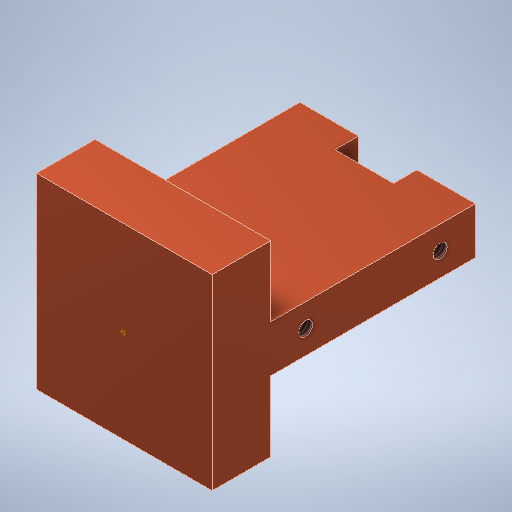
# Autodesk Inventor part: copper_thermal_contact
Saved by Autodesk Inventor 2025 (Build 290162000, 162)
## iProperties
Created: 2024-04-25
Part Number: copper_thermal_contact
Material: Copper
Document SubType Name: Modeling
Designer: warke
Density: 8.94 g/cm^3
Appearance: Copper - Satin
Author: warke
Autodesk Inventor part; units mm, degrees
ref_plane "YZ Plane" through (0, 0, 0) normal (1, 0, 0) x (0, 1, 0)
ref_plane "XZ Plane" through (0, 0, 0) normal (0, 1, 0) x (-1, 0, 0)
ref_plane "XY Plane" through (0, 0, 0) normal (0, 0, 1) x (1, 0, 0)
sketch "Sketch1" plane through (0, 0, 0) normal (0, 1, 0) x (-1, 0, 0)
  line L0 (-7.5, 15) -> (7.5, 15)
  line L1 (7.5, 15) -> (7.5, -15)
  line L2 (7.5, -15) -> (-7.5, -15)
  line L3 (-7.5, -15) -> (-7.5, 15)
  line L4 (-7.5, 15) -> (7.5, -15) construction
  line L5 (7.5, 15) -> (-7.5, -15) construction
  point P0 (0, 0)
  dimension "d0" = 15
  dimension "d1" = 30
  constraints: 12 end point, 2 midpoint, 2 parallel, 1 horizontal, 1 perpendicular
  measures "d0" distance of L1.end L2.end
  measures "d1" distance of L0.end L1.end
extrude "Extrusion1" add sketch "Sketch1" along normal blind 4
chamfer "Chamfer1" distance 2.5 distance2 1 1 edges at (7.5, 2, -15) measured on face at (7.5, 1.3333, 5)
chamfer "Chamfer2" distance 1 distance2 2.5 1 edges at (-7.5, 2, -15) measured on face at (1.8333, 2.6667, -15)
sketch "Sketch3" plane through (0, 0, 0) normal (0, -1, 0) x (1, 0, 0)
  line L0 (0, 0) -> (4, 0)
  line L1 (0, 0) -> (-4, 0)
  dimension "d14" = 4
  dimension "d15" = 4
  constraints: 4 end point, 2 coincident, 2 horizontal
  measures "d14" distance of L0.start L0.end
  measures "d15" distance of L0.start L1.end
hole "Hole1" at (4, 0, 0) at (-4, 0, 0) direction (0, 1, 0) diameter 2.1565 depth 2 thread size "4-40 UNC" class "2B" standard "ANSI Unified Screw Threads"
sketch "Sketch4" plane through (0, 0, 0) normal (0, -1, 0) x (1, 0, 0)
  line L0 (7.5, 15) -> (7.5, -12.5) projected
  line L1 (7.5, -12.5) -> (7.5, -7.5)
  line L2 (7.5, -7.5) -> (2.5, -7.5)
  line L3 (2.5, -7.5) -> (2.5, -5.5)
  line L4 (2.5, -5.5) -> (-2.5, -5.5)
  line L5 (-2.5, -5.5) -> (-2.5, -7.5)
  line L6 (-2.5, -7.5) -> (-7.5679, -7.5)
  line L7 (-7.5679, -7.5) -> (-7.5679, -12.5)
  line L8 (6.5, -15) -> (-6.5, -15) projected
  line L9 (-7.5679, -12.5) -> (-6.5, -15)
  line L10 (7.5, -12.5) -> (6.5, -15) projected
  line L11 (-6.5, -15) -> (6.5, -15)
  line L12 (6.5, -15) -> (7.5, -12.5)
  point P0 (0, 0)
  dimension "d23" = 5
  dimension "d24" = 5
  dimension "d25" = 2
  dimension "d26" = 5
  constraints: 20 end point, 5 perpendicular, 3 point on line, 1 collinear, 1 parallel
  measures "d23" distance of L0.end L1.end
  measures "d24" distance of L1.end L2.end
  measures "d25" distance of L2.end L3.end
  measures "d26" distance of L3.end L4.end
split body "Split1" sketch "Sketch4" result one side removed curves L2 L3 L4 L5 L6 L7 L9 L11 L12 L1 removed pieces at (0.8333, 0.5, -12.5)
sketch "Sketch5" plane through (0, 4, 0) normal (0, 1, 0) x (1, 0, 0)
  line L0 (-7.5, 7.5) -> (-7.5, -15) projected
  line L1 (7.5, -15) -> (7.5, 7.5) projected
  line L2 (-7.5, -15) -> (7.5, -15)
  line L3 (7.5, -15) -> (7.5, -10)
  line L4 (7.5, -10) -> (-7.5, -10)
  line L5 (-7.5, -10) -> (-7.5, -15)
  point P0 (0, 0)
  dimension "d27" = 5
  constraints: 8 end point, 2 parallel, 1 horizontal, 1 perpendicular, 1 point on line
  measures "d27" distance of L3.end L2.end
extrude "Extrusion3" add sketch "Sketch5" along normal blind 6 and the other way blind 10
sketch "Sketch6" plane through (7.5, 0, -7.5) normal (1, 0, 0) x (0, 0, -1)
  line L0 (0, 4) -> (0, 0) projected
  line L1 (0, 2) -> (-3, 2)
  line L2 (-17.5, 2) -> (-14.5, 2)
  point P0 (-7.5, 0)
  dimension "d38" = 3
  dimension "d39" = 3
  constraints: 4 end point, 2 horizontal, 1 midpoint
  measures "d38" distance of L1.start L1.end
  measures "d39" distance of L2.start L2.end
hole "Hole2" at (7.5, 2, 7) at (7.5, 2, -4.5) direction (-1, 0, 0) diameter 1.1811 depth 3 thread size "0-80 UNF" class "2B" standard "ANSI Unified Screw Threads"
sketch "Sketch7" plane through (-7.5, 0, -7.5) normal (-1, 0, 0) x (0, 0, 1)
  circle A0 centre (3, 2) radius 0.5906 projected
  circle A1 centre (14.5, 2) radius 0.5906 projected
  point P0 (7.5, 0)
hole "Hole3" at (-7.5, 2, 7) at (-7.5, 2, -4.5) direction (1, 0, 0) diameter 1.1811 depth 3 thread size "0-80 UNF" class "2B" standard "ANSI Unified Screw Threads"
sketch "Sketch8" plane through (0, -6, 0) normal (0, -1, 0) x (1, 0, 0)
  line L0 (7.5, 10) -> (7.5, 15) projected
  line L1 (7.5, 12.5) -> (4, 12.5)
  line L2 (-7.5, 10) -> (-7.5, 15) projected
  line L3 (-7.5, 12.5) -> (-4, 12.5)
  point P0 (0, 0)
  dimension "d54" = 3.5
  dimension "d55" = 3.5
  constraints: 4 end point, 2 coincident, 2 horizontal, 2 midpoint
  measures "d54" distance of L1.start L1.end
  measures "d55" distance of L3.start L3.end
hole "Hole4" at (4, -6, 12.5) at (-4, -6, 12.5) direction (0, 1, 0) diameter 2.1565 depth 3 thread size "4-40 UNC" class "2B" standard "ANSI Unified Screw Threads"
body "Solid1"
